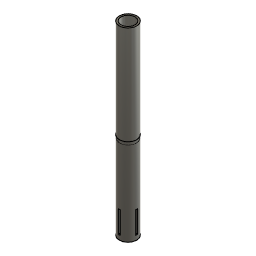
smallRocketBodyTube v2 (Autodesk Fusion 360 design; units mm, degrees)
Autodesk Fusion 360 part; units mm, degrees
sketch "Sketch1" plane through (0, 0, 0) normal (0, 1, 0) x (1, 0, 0)
  circle A0 centre (0, 0) radius 12
  circle A1 centre (0, 0) radius 15
  dimension "d2" = 24
  dimension "d4" = 3
  constraint coincident A0.centre A1.centre
  measures "d2" diameter of A0
extrude "Extrude1" add sketch "Sketch1" along normal blind 320 makes body 1
sketch "Sketch2" plane through (0, 0, 0) normal (1, 0, 0) x (0, 0, -1)
  line L0 (0, 0) -> (0, 8) construction
  line L1 (0, 8) -> (-1.5875, 8)
  line L2 (-1.5875, 8) -> (-1.5875, 46)
  line L3 (-1.5875, 46) -> (0, 46)
  line L4 (0, 8) -> (1.5875, 8)
  line L5 (1.5875, 8) -> (1.5875, 46)
  line L6 (1.5875, 46) -> (0, 46)
  line L7 (0, 46) -> (0, 65) construction
  dimension "d15" = 8
  dimension "d16" = 1.5875
  dimension "d17" = 38
  dimension "d18" = 38
  dimension "d19" = 19
  constraint coincident L0.start origin
  constraint horizontal L1
  constraint vertical L2
  constraint horizontal L3
  constraint horizontal L4
  constraint vertical L5
  constraint horizontal L6
  constraint perpendicular L3 L7
  measures "d15" distance of L0.start L0.end
  measures "d16" distance of L0.end L1.end
  measures "d17" distance of L0.end L3.end
  measures "d18" distance of L0.end L3.end
  measures "d19" distance of L3.end L7.end
sketch "Sketch3" plane through (0, 0, 0) normal (0, 1, 0) x (1, 0, 0)
sketch "Sketch4" plane through (0, 0, 0) normal (0, 1, 0) x (1, 0, 0)
ref_plane "WorkPlane1" through (0, 70, 0) normal (0, 1, 0) x (0, 0, 1)
sketch "Sketch5" plane through (0, 0, 0) normal (1, 0, 0) x (0, 0, -1)
extrude "Extrude2" cut sketch "Sketch2" along normal blind 19 and the other way blind 18 bodies 1
sketch "Sketch6" plane through (0, 0, 0) normal (0, 1, 0) x (1, 0, 0)
sketch "Sketch7" plane through (0, 0, 0) normal (0, 0, 1) x (1, 0, 0)
  line L0 (0, 0) -> (0, 8) construction
  line L1 (0, 8) -> (1.5875, 8)
  line L2 (1.5875, 8) -> (1.5875, 46)
  line L3 (1.5875, 46) -> (0, 46)
  line L4 (0, 8) -> (-1.5875, 8)
  line L5 (-1.5875, 8) -> (-1.5875, 46)
  line L6 (-1.5875, 46) -> (0, 46)
  line L7 (0, 46) -> (0, 65) construction
  dimension "d24" = 8
  dimension "d25" = 1.5875
  dimension "d26" = 38
  dimension "d27" = 38
  dimension "d28" = 19
  constraint coincident L0.start origin
  constraint vertical L0
  constraint horizontal L1
  constraint vertical L2
  constraint horizontal L3
  constraint horizontal L4
  constraint vertical L5
  constraint horizontal L6
  constraint perpendicular L6 L7
  measures "d24" distance of L0.start L0.end
  measures "d25" distance of L0.end L1.end
  measures "d26" distance of L0.end L3.end
  measures "d27" distance of L0.end L3.end
  measures "d28" distance of L3.end L7.end
extrude "Extrude3" cut sketch "Sketch7" along normal mid plane 36 bodies 1
ref_plane "WorkPlane2" through (0, 150, 0) normal (0, 1, 0) x (0, 0, 1)
split "Split1" by plane through (0, 150, 0) normal (0, 1, 0) bodies 1 makes body 2 at (14.9255, 206.6667, -1.4935)
sketch "Sketch8" plane through (0, 0, 0) normal (0, 0, 1) x (1, 0, 0)
ref_plane "WorkPlane3" through (0, 12.125, 0) normal (0.707107, 0, 0.707107) x (0, 1, 0)
sketch "Sketch9" plane through (0, 12.125, 0) normal (0.707107, 0, 0.707107) x (0, 1, 0)
sketch "Sketch10" plane through (0, 12.125, 0) normal (0.707107, 0, 0.707107) x (0, 1, 0)
sketch "Sketch11" plane through (0, 12.125, 0) normal (0.707107, 0, 0.707107) x (0, 1, 0)
sketch "Sketch12" plane through (0, 12.125, 0) normal (0.707107, 0, 0.707107) x (0, 1, 0)
sketch "Sketch13" plane through (0, 12.125, 0) normal (0.707107, 0, 0.707107) x (0, 1, 0)
sketch "Sketch14" plane through (0, 12.125, 0) normal (0.707107, 0, 0.707107) x (0, 1, 0)
sketch "Sketch15" plane through (0, 150, 0) normal (0, 1, 0) x (-1, 0, 0)
  circle A0 centre (0, 0) radius 12
  circle A1 centre (0, 0) radius 15
  circle A2 centre (0, 0) radius 12.75
  circle A3 centre (0, 0) radius 14.25
  dimension "d33" = 0.75
  dimension "d34" = -0.75
extrude "Extrude4" cut sketch "Sketch15" against normal blind 5 contours A3 bodies 1
sketch "Sketch16" plane through (0, 150, 0) normal (0, -1, 0) x (1, 0, 0)
  circle A0 centre (0, 0) radius 15
  circle A1 centre (0, 0) radius 12
  circle A2 centre (0, 0) radius 12.753
  circle A3 centre (0, 0) radius 14.247
  dimension "d37" = 0.753
  dimension "d38" = -0.753
extrude "Extrude5" add sketch "Sketch16" along normal blind 5 contours A3 bodies 2
copy_body "Body->Comp1" bodies 1 removing the originals makes body 3 in component "Component"
copy_body "Body->Comp2" bodies 2 removing the originals makes body 4 in component "Component'"
component "Component" placed x (1, 0, 0) y (0, 1, 0) z (0, 0, 1) at (0, 0, 0)
component "Component'" placed x (1, 0, 0) y (0, 1, 0) z (0, 0, 1) at (0, 0, 0)
equation "innerDiameter = 24 mm"
equation "thickness = 3 mm"
equation "d4 = thickness"
equation "length = 320 mm"
equation "d6 = length"
equation "finLength = 50 mm"
equation "finWidth = 0.125 in"
equation "d16 = finWidth / 2"
equation "d25 = finWidth / 2"
